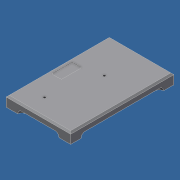
# Autodesk Inventor part: Grundplatte
Saved by Autodesk Inventor 2018 (Build 220112000, 112)
## iProperties
Created: 2018-09-04
Part Number: Grundplatte
Material: Generisch
Document SubType Name: Modeling
Designer: M.Knabel
Density: 1 g/cm^3
Appearance: Vorgabe
Author: M.Knabel
Autodesk Inventor part; units mm, degrees
ref_plane "YZ Plane" through (0, 0, 0) normal (1, 0, 0) x (0, 1, 0)
ref_plane "XZ Plane" through (0, 0, 0) normal (0, 1, 0) x (-1, 0, 0)
ref_plane "XY Plane" through (0, 0, 0) normal (0, 0, 1) x (1, 0, 0)
sketch "Skizze1" plane through (0, 0, 0) normal (0, 0, 1) x (1, 0, 0)
  line L0 (-87.5, 0) -> (87.5, 0) projected
  line L1 (0, -140) -> (0, 140) projected
  line L2 (-62.5, 100) -> (62.5, 100)
  line L3 (62.5, 100) -> (62.5, -100)
  line L4 (62.5, -100) -> (-62.5, -100)
  line L5 (-62.5, -100) -> (-62.5, 100)
  point P0 (0, 0)
  dimension "d0" = 125
  dimension "d1" = 200
  constraints: 8 end point, 2 parallel, 1 perpendicular, 2 other
  measures "d0" distance between parallel lines of L3 L5
  measures "d1" distance between parallel lines of L4 L2
extrude "Grundkörper" add sketch "Skizze1" along normal blind 20
chamfer "umlaufende Fase 3x45°" distance 3 angle 45 4 edges at (0, -100, 20) (62.5, 0, 20) (0, 100, 20) (-62.5, 0, 20)
sketch "Fräsung Rund" plane through (-62.5, -100, 0) normal (0, -1, 0) x (1, 0, 0)
  line L0 (62.5, -4) -> (62.5, 24) projected
  line L1 (-25, 0) -> (150, 0) projected
  line L2 (125, 0) -> (0, 0) projected
  line L3 (30.5, 8) -> (94.5, 8)
  arc A0 (102.5, 0) -> (94.5, 8) centre (94.5, 0) ccw
  arc A1 (30.5, 8) -> (22.5, 0) centre (30.5, 0) ccw
  point P0 (62.5, 0)
  dimension "d13" = 80
  dimension "d14" = 8
  dimension "d15" = 8
  dimension "d16" = 8
  constraints: 4 point on circle, 4 point on line, 2 centre point, 2 end point, 1 horizontal, 1 symmetric about line
  measures "d13" distance of A0.start A1.end
  measures "d14" distance between parallel lines of L1 L3
  measures "d15" radius of A1
  measures "d16" radius of A0
extrude "Querfräsung 80" cut sketch "Fräsung Rund" against normal blind 8
fillet "Rundung Querfräsung" radius 8 3 edges at (37.6569, -92, 5.6569) (-37.6569, -92, 5.6569) (0, -92, 8)
mirror "Spiegeln Querfräsung" about plane through (0, 0, 0) normal (0, 1, 0) of "Querfräsung 80", "Rundung Querfräsung"
sketch "Skizze5" plane through (62.5, -100, 0) normal (1, 0, 0) x (0, 0, -1)
  line L0 (0, -40) -> (0, 240) projected
  line L1 (4, 100) -> (-24, 100) projected
  line L2 (0, 200) -> (0, 0) projected
  arc A0 (-8, 28) -> (0, 20) centre (0, 28) ccw
  arc A1 (0, 180) -> (-8, 172) centre (0, 172) ccw
  line L3 (-8, 28) -> (-8, 172)
  point P0 (0, 100)
  dimension "d21" = 8
  dimension "d22" = 8
  dimension "d23" = 8
  dimension "d24" = 160
  constraints: 4 point on circle, 4 point on line, 2 centre point, 2 end point, 1 parallel, 1 symmetric about line
  measures "d21" distance between parallel lines of L0 L3
  measures "d22" radius of A1
  measures "d23" radius of A0
  measures "d24" distance of A1.start A0.end
extrude "Längsfräsung 160" cut sketch "Skizze5" against normal blind 8
fillet "Rundung Längsfräsung" radius 8 3 edges at (54.5, 77.6569, 5.6569) (54.5, -77.6569, 5.6569) (54.5, 0, 8)
mirror "Spiegeln Längsfräsung" about plane through (0, 0, 0) normal (1, 0, 0) of "Längsfräsung 160", "Rundung Längsfräsung"
sketch "Skizze6" plane through (0, 0, 20) normal (0, 0, 1) x (1, 0, 0)
  line L0 (-87.5, 0) -> (87.5, 0) projected
  line L1 (0, -140) -> (0, 140) projected
  line L2 (-54.5, -20) -> (-35.5, -20)
  line L3 (-35.5, -20) -> (-35.5, 20)
  line L4 (-35.5, 20) -> (-54.5, 20)
  line L5 (-54.5, 20) -> (-54.5, -20)
  line L6 (-62.5, 100) -> (-62.5, -100) projected
  point P0 (0, 0)
  dimension "d28" = 19
  dimension "d29" = 40
  dimension "d34" = 8
  constraints: 8 end point, 2 parallel, 1 horizontal, 1 perpendicular, 1 other
  measures "d28" distance between parallel lines of L3 L5
  measures "d29" distance between parallel lines of L4 L2
  measures "d34" distance between parallel lines of L6 L5
extrude "Tasche 40x19x1,2" cut sketch "Skizze6" against normal blind 1.2
fillet "Rundung Tasche" radius 2 4 edges at (-54.5, 20, 19.4) (-54.5, -20, 19.4) (-35.5, 20, 19.4) (-35.5, -20, 19.4)
sketch "Skizze9" plane through (0, 0, 0) normal (0, 0, -1) x (-1, 0, 0)
  line L0 (-62.5, -100) -> (-40, -100) projected
  line L1 (0, -140) -> (0, 140) projected
  line L2 (87.5, 0) -> (-87.5, 0) projected
  line L3 (62.5, -100) -> (62.5, -80) projected
  line L4 (40, -100) -> (62.5, -100) projected
  point P0 (0, 0)
  point P1 (21.5, -66.5)
  point P2 (0, 28)
  dimension "d65" = 33.5
  dimension "d66" = 94.5
  dimension "d67" = 21.5
  constraints: 1 point on line
  measures "d65" distance from line of L4 point (21.5, -66.5)
  measures "d66" vertical distance of point (0, 28) point (21.5, -66.5)
  measures "d67" distance from line of L1 point (21.5, -66.5)
hole "Durchgangsbohrung Ø4,5" at (-21.5, -66.5, 0) at (0, 28, 0) direction (0, 0, 1) diameter 4.5 end through all counterbore diameter 8 counterbore depth 4.6 clearance for "Sechskantkopfschraube DIN EN 24017" size "M4" standard "DIN"
sketch "Skizze10" plane through (0, 0, 0) normal (0, 0, -1) x (-1, 0, 0)
  line L0 (-32, 100) -> (32, 100) projected
  line L1 (62.5, 72) -> (62.5, -72) projected
  line L2 (-87.5, 0) -> (87.5, 0) projected
  line L3 (0, -140) -> (0, 140) projected
  circle A0 centre (-50, 88) radius 5
  circle A1 centre (50, 88) radius 5
  circle A2 centre (-50, -88) radius 5
  circle A3 centre (50, -88) radius 5
  point P0 (0, 0)
  dimension "d68" = 50
  dimension "d69" = 100
  dimension "d70" = 176
  dimension "d71" = 176
  dimension "d72" = 50
  dimension "d73" = 100
  dimension "d74" = 10
  dimension "d75" = 10
  dimension "d76" = 10
  dimension "d77" = 10
  constraints: 4 centre point, 1 symmetric about line
  measures "d68" distance from line of L3 A0.centre
  measures "d69" distance of A1.centre A0.centre
  measures "d70" distance of A3.centre A1.centre
  measures "d71" distance of A2.centre A0.centre
  measures "d72" distance from line of L3 A2.centre
  measures "d73" distance of A3.centre A2.centre
  measures "d74" diameter of A3
  measures "d75" diameter of A2
  measures "d76" diameter of A0
  measures "d77" diameter of A1
extrude "Extrusion5" cut sketch "Skizze10" against normal blind 2
